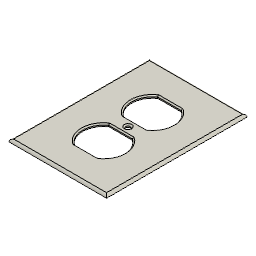
OutletCover (Autodesk Fusion 360 design; units mm, degrees)
part number: 2026-06-18-11-25-44-078
Autodesk Fusion 360 part; units mm, degrees
sketch "Sketch1" plane through (0, 0, 0) normal (0, 0, 1) x (1, 0, 0)
  line L0 (40, -57.5) -> (40, 57.5)
  line L1 (40, 57.5) -> (-40, 57.5)
  line L2 (40, -57.5) -> (-40, -57.5)
  line L3 (-40, -57.5) -> (-40, 57.5)
  circle A0 centre (0, 0) radius 2
  line L4 (40, 57.5) -> (-40, -57.5) construction
  line L5 (-9.6437, 34) -> (9.6437, 34)
  line L6 (9.6437, 36.1637) -> (9.6437, 6) construction
  line L7 (9.6437, 6) -> (-9.6437, 6)
  line L8 (-9.6437, 6) -> (-9.6437, 34) construction
  line L9 (9.6437, -6) -> (-9.6437, -6)
  line L10 (-9.6437, -6) -> (-9.6437, -34) construction
  line L11 (-9.6437, -34) -> (9.6437, -34)
  line L12 (9.6437, -34) -> (9.6437, -6) construction
  line L13 (-40, 0) -> (40, 0) construction
  line L14 (0, 34) -> (0, 57.5)
  arc A1 (-9.6437, 34) -> (-9.6437, 6) centre (0, 20) ccw
  arc A2 (9.6437, 6) -> (9.6437, 34) centre (0, 20) ccw
  arc A3 (9.6437, -34) -> (9.6437, -6) centre (0, -20) ccw
  arc A4 (-9.6437, -6) -> (-9.6437, -34) centre (0, -20) ccw
  dimension "d1" = 4
  dimension "d2" = 17
  dimension "d3" = 115
  dimension "d4" = 80
  dimension "d6" = 28
  dimension "d8" = 6
  constraint coincident L1.end L3.end
  constraint coincident L0.start L2.start
  constraint perpendicular L0 L1
  constraint vertical L0
  constraint vertical L3
  constraint horizontal L2
  constraint midpoint A0.centre L4
  constraint horizontal L5
  constraint vertical L6
  constraint horizontal L7
  constraint vertical L8
  constraint horizontal L9
  constraint vertical L10
  constraint horizontal L11
  constraint vertical L12
  constraint midpoint L0 L13.end
  constraint midpoint L3 L13.start
  constraint symmetric L8 L10 L13
  constraint symmetric L7 L9 L13
  constraint symmetric L5 L11 L13
  constraint midpoint L5 L14.start
  constraint midpoint L1 L14.end
  constraint equal A1 A2
  constraint equal A3 A4
  constraint equal A1 A4
  constraint coincident A0.centre origin
  constraint coincident L5.end A2.end
  constraint concentric A1 A2
  constraint vertical L14
  measures "d1" diameter of A0
  measures "d2" radius of A1
  measures "d3" distance of L2.end L1.end
  measures "d4" distance of L0.end L1.end
  measures "d6" distance of L5 L7
  measures "d8" distance of L7 L13
extrude "Extrude1" add sketch "Sketch1" along normal blind 2
fillet "Fillet1" radius 2 4 edges at (0, 57.5, 2) (-40, 0, 2) (0, -57.5, 2) (40, 0, 2)
fillet "Fillet2" radius 1 8 edges at (17, -20, 2) (0, -6, 2) (-17, -20, 2) (0, -34, 2) (17, 20, 2) (0, 6, 2) (-17, 20, 2) (0, 34, 2)
chamfer "Chamfer1" distance 1 angle 45 1 edges at (-1.8647, 0.7232, 2)
